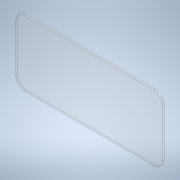
# Autodesk Inventor part: Wind Tunnel Test Section Door Inner
Saved by Autodesk Inventor 2020 (Build 240168000, 168)
## iProperties
Created: 2022-03-09
Part Number: Wind Tunnel Test Section Door Inner
Material: Polycarbonate, Clear
Document SubType Name: Modeling
Designer: kamer
Density: 1.2 g/cm^3
Appearance: Polycarbonate - Clear
Author: kamer
Autodesk Inventor part; units mm, degrees
ref_plane "YZ Plane" through (0, 0, 0) normal (1, 0, 0) x (0, 1, 0)
ref_plane "XZ Plane" through (0, 0, 0) normal (0, 1, 0) x (-1, 0, 0)
ref_plane "XY Plane" through (0, 0, 0) normal (0, 0, 1) x (1, 0, 0)
sketch "Sketch1" plane through (0, 0, 0) normal (0, 0, 1) x (1, 0, 0)
  line L0 (25.4, 0) -> (430.0474, 0)
  line L1 (455.4474, 25.4) -> (455.4474, 179.3494)
  line L2 (430.0474, 204.7494) -> (25.4, 204.7494)
  line L3 (0, 179.3494) -> (0, 25.4)
  arc A0 (25.4, 204.7494) -> (0, 179.3494) centre (25.4, 179.3494) ccw
  arc A1 (455.4474, 179.3494) -> (430.0474, 204.7494) centre (430.0474, 179.3494) ccw
  arc A2 (430.0474, 0) -> (455.4474, 25.4) centre (430.0474, 25.4) ccw
  arc A3 (0, 25.4) -> (25.4, 0) centre (25.4, 25.4) ccw
  point P0 (0, 0)
  point P1 (455.4474, 204.7494)
  point P2 (0, 204.7494)
  dimension "d0" = 455.4474
  dimension "d1" = 204.7494
  dimension "d2" = 25.4
  constraints: 8 end point, 8 point on circle, 8 tangent, 6 point on line, 4 centre point, 3 equal radius, 2 parallel, 1 horizontal, 1 perpendicular
  measures "d0" distance of point (455.447, 204.749) point (0, 204.749)
  measures "d1" distance between parallel lines of L0 L2
  measures "d2" radius of A0
extrude "Extrusion1" add sketch "Sketch1" along normal blind 5.7658
body "Solid1"
